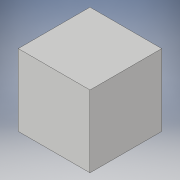
# Autodesk Inventor part: Hydraulic tank
Saved by Autodesk Inventor 2019 (Build 230136000, 136)
## iProperties
Created: 2020-10-19
Part Number: Hydraulic tank
Material: Generic
Document SubType Name: Modeling
Designer: Jawal
Density: 1 g/cm^3
Appearance: Default
Author: Jawal
Autodesk Inventor part; units mm, degrees
ref_plane "YZ Plane" through (0, 0, 0) normal (1, 0, 0) x (0, 1, 0)
ref_plane "XZ Plane" through (0, 0, 0) normal (0, 1, 0) x (-1, 0, 0)
ref_plane "XY Plane" through (0, 0, 0) normal (0, 0, 1) x (1, 0, 0)
sketch "Sketch1" plane through (0, 0, 0) normal (0, 0, 1) x (1, 0, 0)
  line L0 (-98, -98) -> (98, -98)
  line L1 (98, -98) -> (98, 98)
  line L2 (98, 98) -> (-98, 98)
  line L3 (-98, 98) -> (-98, -98)
  line L4 (-98, -98) -> (98, 98) construction
  line L5 (98, -98) -> (-98, 98) construction
  point P0 (0, 0)
  dimension "d0" = 196
  dimension "d1" = 196
  constraints: 12 end point, 2 midpoint, 2 parallel, 1 horizontal, 1 perpendicular
  measures "d0" distance of L2.end L1.end
  measures "d1" distance of L1.end L0.end
extrude "Extrusion1" add sketch "Sketch1" along normal blind 196
body "Solid1"
